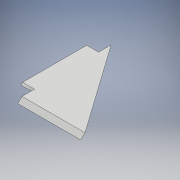
# Autodesk Inventor part: Rooft Extension Right Attachment
Saved by Autodesk Inventor 2017 (Build 210142000, 142)
## iProperties
Created: 2018-03-30
Part Number: Rooft Extension Right Attachment
Material: Generic
Document SubType Name: Modeling
Designer: Arjuna
Density: 1 g/cm^3
Appearance: Default
Author: Arjuna
## iProperties of the stored document Roof Extension Right Attachment_3DPrint.ipt
Created: 2018-03-30
Part Number: Roof Extension Right Attachment_3DPrint
Material: Generic
Document SubType Name: Modeling
Designer: Arjuna
Density: 1 g/cm^3
Appearance: Default
Author: Arjuna
Autodesk Inventor part; units mm, degrees
ref_plane "YZ Plane" through (0, 0, 0) normal (1, 0, 0) x (0, 1, 0)
ref_plane "XZ Plane" through (0, 0, 0) normal (0, 1, 0) x (-1, 0, 0)
ref_plane "XY Plane" through (0, 0, 0) normal (0, 0, 1) x (1, 0, 0)
sketch "Sketch1" plane through (0, 0, 0) normal (0, 0, 1) x (1, 0, 0)
  line L0 (0, 8.9862) -> (0, -66.0138)
  line L1 (0, 8.9862) -> (53, -66.0138)
  line L2 (0, -66.0138) -> (53, -66.0138)
  point P0 (0, 0)
  dimension "d0" = 75
  dimension "d39" = 53
  constraints: 6 end point, 1 horizontal, 1 vertical
  measures "d0" distance of L0.start L0.end
  measures "d39" distance of L0.end L1.end
sketch "Sketch2" plane through (0, 0, 0) normal (1, 0, 0) x (0, 1, 0)
  line L0 (4.5625, 0) -> (1.027, -3.5355)
  line L1 (1.9119, 0) -> (-2.0934, 0)
  point P0 (0, 0)
  dimension "d2" = 45
  dimension "d3" = 5
  constraints: 4 end point, 1 horizontal
  measures "d2" angle of L1 L0
  measures "d3" distance of L0.start L0.end
sweep "Sweep1" add profiles "Sketch1" path "Sketch2" path curves L0
sketch "Sketch3" plane through (0, -66.0138, 0) normal (-1, 0, 0) x (0, 0, 1)
  line L0 (0, 75) -> (0, 0) projected
  line L1 (0, 75) -> (-3.5355, 71.4645) projected
  line L2 (-3.5355, -3.5355) -> (-3.5355, 71.4645) projected
  line L3 (0, 0) -> (-3.5355, -3.5355) projected
  line L4 (0, 64.5) -> (-1.4142, 63.0858)
  line L5 (-1.4142, 63.0858) -> (-1.4142, 9.0858)
  line L6 (-1.4142, 9.0858) -> (0, 10.5)
  point P0 (0, 66.0138)
  dimension "d6" = 2
  dimension "d7" = 2
  dimension "d8" = 54
  dimension "d9" = 75
  dimension "d10" = 10.5
  dimension "d11" = 10.5
  constraints: 6 end point, 2 parallel, 2 point on line
  measures "d6" distance of L4.end L4.start
  measures "d7" distance of L5.end L6.end
  measures "d8" distance of L5.end L4.end
  measures "d9" distance of L0.start L0.end
  measures "d10" distance of L4.start L0.start
  measures "d11" distance of L0.end L6.end
extrude "Extrusion1" add sketch "Sketch3" along normal blind 10 contours L0 L6 L5 L4
sketch "Sketch5" plane through (0, -56.9281, -1.4142) normal (0, 0, -1) x (-1, 0, 0)
  line L0 (0, 0) -> (0, 54) projected
  line L1 (0, 0) -> (10, 0) projected
  line L2 (10, 54) -> (10, 0) projected
  line L3 (0, 54) -> (10, 54) projected
  line L4 (4.25, 45.5) -> (6.25, 45.5)
  line L5 (6.25, 45.5) -> (6.25, 31.5)
  line L6 (6.25, 31.5) -> (4.25, 31.5)
  line L7 (4.25, 31.5) -> (4.25, 45.5)
  line L8 (4.25, 22.5) -> (6.25, 22.5)
  line L9 (6.25, 22.5) -> (6.25, 8.5)
  line L10 (6.25, 8.5) -> (4.25, 8.5)
  line L11 (4.25, 8.5) -> (4.25, 22.5)
  point P0 (0, 56.9281)
  dimension "d28" = 2
  dimension "d29" = 8.5
  dimension "d30" = 4.25
  dimension "d31" = 14
  dimension "d32" = 14
  dimension "d33" = 8.5
  dimension "d34" = 9
  dimension "d35" = 54
  constraints: 16 end point, 4 parallel, 2 horizontal, 2 perpendicular, 2 point on line
  measures "d28" distance between parallel lines of L5 L7
  measures "d29" distance between parallel lines of L4 L3
  measures "d30" distance from line of L0 L4.start
  measures "d31" distance of L4.end L5.end
  measures "d32" distance between parallel lines of L10 L8
  measures "d33" distance between parallel lines of L1 L10
  measures "d34" distance from line of L8.end L6
  measures "d35" distance of L2.start L1.end
sketch "Sketch6" plane through (0, -69.5494, -3.5355) normal (-1, 0, 0) x (0, 0, 1)
  line L0 (3.5355, 14.0355) -> (2.1213, 12.6213) projected
  line L1 (2.1213, 12.6213) -> (2.1213, 66.6213) projected
  line L2 (2.1213, 66.6213) -> (3.5355, 68.0355) projected
  line L3 (3.5355, 78.5355) -> (3.5355, 68.0355) projected
  line L4 (3.5355, 78.5355) -> (0, 75) projected
  line L5 (0, 0) -> (0, 75) projected
  line L6 (3.5355, 3.5355) -> (0, 0) projected
  line L7 (3.5355, 14.0355) -> (3.5355, 3.5355) projected
  line L8 (3.5355, 68.0355) -> (2.1213, 66.6213) projected
  line L9 (2.1213, 66.6213) -> (2.1213, 12.6213) projected
  line L10 (2.1213, 12.6213) -> (3.5355, 14.0355) projected
  line L11 (3.5355, 14.0355) -> (3.5355, 68.0355) projected
  line L12 (2.1213, 64.596) -> (-1.4142, 61.0605)
  point P0 (3.5355, 69.5494)
  dimension "d36" = 5
  constraints: 2 end point, 1 point on line
  measures "d36" distance of L12.start L12.end
sweep "Sweep2" add profiles "Sketch5" path "Sketch6" path curves L12 contours L4 L5 L6 L7 | L8 L9 L10 L11
equation "\"d10\" = -0.5 * d8 + 0.5 * d9"
equation "\"d32\" = d31"
equation "\"d33\" = d29"
body "Solid1"
